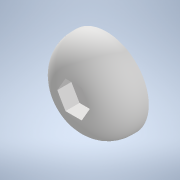
# Autodesk Inventor part: ENDER 3 E_PLATE_SCREW
Saved by Autodesk Inventor 2022 (Build 260153070, 153G)
## iProperties
Created: 2022-01-01
Part Number: ENDER 3 E_PLATE_SCREW
Material: Generic
Document SubType Name: Modeling
Designer: a laptop
Density: 1 g/cm^3
Appearance: Default
Author: a laptop
Autodesk Inventor part; units mm, degrees
ref_plane "YZ Plane" through (0, 0, 0) normal (1, 0, 0) x (0, 1, 0)
ref_plane "XZ Plane" through (0, 0, 0) normal (0, 1, 0) x (-1, 0, 0)
ref_plane "XY Plane" through (0, 0, 0) normal (0, 0, 1) x (1, 0, 0)
sketch "Sketch1" plane through (0, 0, 0) normal (0, 0, 1) x (1, 0, 0)
  circle A0 centre (0, 0) radius 4.5
  dimension "d0" = 9
  constraints: 1 centre point, 1 coincident
  measures "d0" diameter of A0
extrude "Extrusion1" add sketch "Sketch1" along normal blind 3.5
fillet "Fillet1" radius 3 1 edges at (-4.5, 0, 3.5)
sketch "Sketch2" plane through (0, 0, 3.5) normal (0, 0, 1) x (1, 0, 0)
  line L0 (1.7321, 0) -> (0.866, -1.5)
  line L1 (0.866, -1.5) -> (-0.866, -1.5)
  line L2 (-0.866, -1.5) -> (-1.7321, 0)
  line L3 (-1.7321, 0) -> (-0.866, 1.5)
  line L4 (-0.866, 1.5) -> (0.866, 1.5)
  line L5 (0.866, 1.5) -> (1.7321, 0)
  point P0 (0, 0)
  point P1 (0, 0)
  dimension "d4" = 3
  constraints: 12 end point, 1 coincident, 1 horizontal, 13 other
  measures "d4" distance between parallel lines of L1 L4
extrude "Extrusion2" cut sketch "Sketch2" against normal blind 1.5
body "Solid1"
